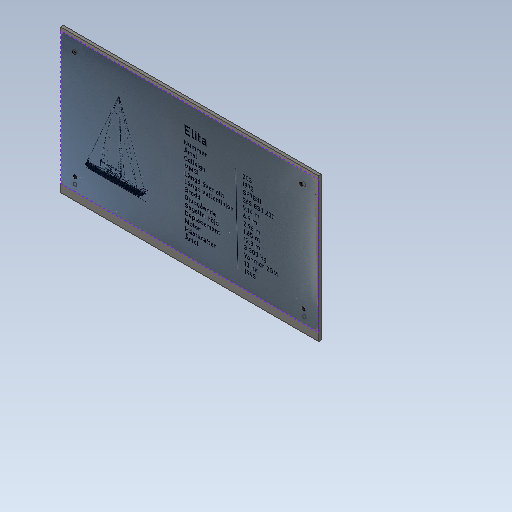
# Autodesk Inventor part: infosign
Saved by Autodesk Inventor 2021 (Build 250183000, 183)
## iProperties
Created: 2020-05-19
Part Number: infosign
Material: Stainless Steel
Document SubType Name: Modeling
Designer: Johansson
Density: 8 g/cm^3
Appearance: Semi-Polished
Author: Johansson
Autodesk Inventor part; units mm, degrees
ref_plane "YZ Plane" through (0, 0, 0) normal (1, 0, 0) x (0, 1, 0)
ref_plane "XZ Plane" through (0, 0, 0) normal (0, 1, 0) x (-1, 0, 0)
ref_plane "XY Plane" through (0, 0, 0) normal (0, 0, 1) x (1, 0, 0)
sketch "Sketch1" plane through (0, 0, 0) normal (0, 0, 1) x (1, 0, 0)
  line L0 (-90, -50) -> (90, -50)
  line L1 (90, -50) -> (90, 50)
  line L2 (90, 50) -> (-90, 50)
  line L3 (-90, 50) -> (-90, -50)
  line L4 (-90, -50) -> (90, 50) construction
  line L5 (90, -50) -> (-90, 50) construction
  point P0 (0, 0)
  dimension "d0" = 180
  dimension "d1" = 100
  constraints: 12 end point, 2 midpoint, 2 parallel, 1 horizontal, 1 perpendicular
  measures "d0" distance of L1.end L2.end
  measures "d1" distance of L0.end L1.end
extrude "Extrusion1" add sketch "Sketch1" along normal blind 2
sketch "Sketch2" plane through (0, 0, 2) normal (0, 0, 1) x (1, 0, 0)
  line L0 (-89.9951, 47.8948) -> (90.667, 47.8948) construction
  line L1 (90.667, 47.8948) -> (90.667, -44.4596) construction
  line L2 (90.667, -44.4596) -> (-89.9951, -44.4596) construction
  line L3 (-89.9951, -44.4596) -> (-89.9951, 47.8948) construction
  constraints: 2 other
sketch "Sketch3" plane through (0, 0, 2) normal (0, 0, 1) x (1, 0, 0)
  circle A0 centre (-80, 40) radius 1.25
  line L0 (-126.1334, 0) -> (126.8004, 0) projected
  line L1 (0, -70) -> (0, 70) projected
  circle A1 centre (80, 40) radius 1.25
  circle A2 centre (-80, -40) radius 1.25
  circle A3 centre (80, -40) radius 1.25
  line L2 (90, 50) -> (-90, 50) projected
  line L3 (-90, 50) -> (-90, -50) projected
  point P0 (0, 0)
  dimension "d21" = 2.5
  dimension "d23" = 10
  dimension "d24" = 10
  constraints: 4 centre point, 3 symmetric about line, 3 other
  measures "d21" diameter of A0
  measures "d23" distance from line of A0.centre L2
  measures "d24" distance from line of A0.centre L3
extrude "Extrusion2" cut sketch "Sketch3" against normal up to next contours A0 | A1 | A2 | A3
equation "\"d0\" = l_infosign"
equation "\"d1\" = w_infosign"
equation "\"wl_panel\" = 285"
equation "\"t_panel\" = 8"
equation "\"r_button\" = 8"
equation "\"l_stereo\" = 178"
equation "\"d_stereo\" = 177"
equation "\"w_label\" = 15"
equation "\"r_labelscrew\" = 2.5"
equation "\"ro_labelscrew\" = 5"
equation "\"l_buttontobutton\" = 25"
equation "\"r_usboutlet\" = 29"
equation "\"l_fastener_button\" = 19"
equation "\"w_infosign\" = 100"
equation "\"l_infosign\" = 180"
body "Solid1"
